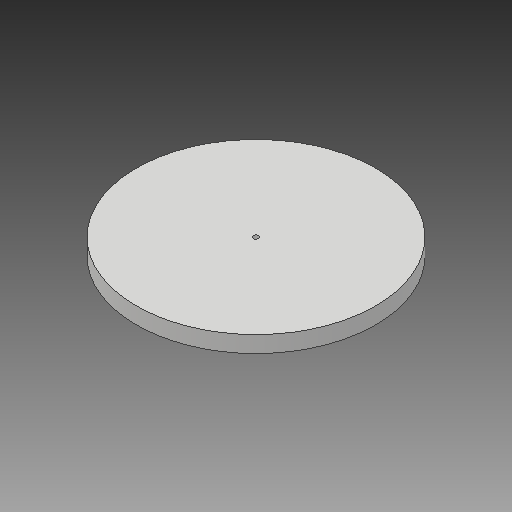
# Autodesk Inventor part: Rueda Interna
Saved by Autodesk Inventor 2017 (Build 210142000, 142)
## iProperties
Created: 2017-01-19
Part Number: Rueda Interna
Material: Generic
Document SubType Name: Modeling
Designer: A. Matías Quezada
Density: 1 g/cm^3
Appearance: Default
Author: A. Matías Quezada
Autodesk Inventor part; units mm, degrees
ref_plane "YZ Plane" through (0, 0, 0) normal (1, 0, 0) x (0, 1, 0)
ref_plane "XZ Plane" through (0, 0, 0) normal (0, 1, 0) x (-1, 0, 0)
ref_plane "XY Plane" through (0, 0, 0) normal (0, 0, 1) x (1, 0, 0)
sketch "Sketch1" plane through (0, 0, 0) normal (0, 0, 1) x (1, 0, 0)
  circle A0 centre (0, 0) radius 21.8
  dimension "d0" = 43.6
  constraints: 1 centre point, 1 coincident
  measures "d0" diameter of A0
extrude "Cuerpo" add sketch "Sketch1" along normal blind 3
sketch "Sketch2" plane through (0, 0, 0) normal (0, 0, -1) x (-1, 0, 0)
  circle A0 centre (0, 14.3) radius 5
  point P0 (0, 0)
  dimension "d4" = 14.3
  dimension "d5" = 10
  constraints: 1 centre point, 1 coincident
  measures "d4" distance of point (0, 0) point (0, 14.3)
  measures "d5" diameter of A0
extrude "Manivela" add sketch "Sketch2" along normal blind 3
sketch "Sketch3" plane through (0, 0, 0) normal (0, 0, -1) x (-1, 0, 0)
  circle A0 centre (0, 0) radius 21.8 projected
  constraints: 1 coincident
hole "Centro" at (0, 0, 0) direction (0, 0, 1) diameter 1 end through all
equation "\"d0\" = ri_diametro"
equation "\"d1\" = ri_grosor"
equation "\"d4\" = ri_eje_separacion"
equation "\"d5\" = ri_eje_diametro"
equation "\"d6\" = ri_eje_grosor"
equation "\"d8\" = ri_ancla_diametro"
equation "\"ri_diametro\" = 43.6"
equation "\"ri_grosor\" = 3"
equation "\"ri_eje_diametro\" = 10"
equation "\"ri_eje_grosor\" = 3"
equation "\"ri_ancla_diametro\" = 1"
equation "\"ri_eje_separacion\" = 14.3"
body "Solid1"
